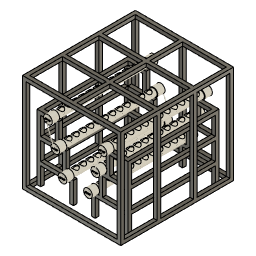
시설 스마트팜 도면 (Autodesk Fusion 360 design; units mm, degrees)
Autodesk Fusion 360 part; units mm, degrees
note: some values were not read from the file. Set by a fixed rule: which face or edge a step refers to.
sketch "스케치1" plane through (0, 0, 0) normal (0, 1, 0) x (1, 0, 0)
  line L0 (0, 0) -> (0, -100)
  line L1 (0, -100) -> (5, -100)
  line L2 (5, -100) -> (5, 0)
  line L3 (5, 0) -> (0, 0)
  dimension "d1" = 100
  dimension "d2" = 5
  constraint vertical L0
  constraint coincident L0.start L3.end
  constraint perpendicular L0 L1
  constraint perpendicular L1 L2
  constraint perpendicular L0 L3
  measures "d1" distance of L0.start L0.end
  measures "d2" distance of L0.end L1.end
extrude "돌출1" add sketch "스케치1" along normal blind 5 makes body 1
copy_body "CopyPasteBodies1" bodies 1 makes body 2
move_body "이동1" bodies 2 to x (1, 0, 0) y (0, 1, 0) z (0, 0, 1) at (70, 0, 0)
copy_body "CopyPasteBodies2" bodies 1 makes body 3
move_body "이동2" bodies 3 to x (0, 0, 1) y (0, 1, 0) z (-1, 0, 0) at (100, 0, 100)
extrude "돌출2" cut 1 faces at (100, 1.6667, 103.3333) along direction (-1, 0, 0) blind 25 on bodies 3 bodies 3
copy_body "CopyPasteBodies3" bodies 1 2 3 makes body 4 makes body 5 makes body 6
move_body "이동3" bodies 4 5 6 to x (1, 0, 0) y (0, 1, 0) z (0, 0, 1) at (0, 50, 0)
copy_body "CopyPasteBodies4" bodies 4 6 5 makes body 7 makes body 8 makes body 9
move_body "이동4" bodies 7 8 9 to x (1, 0, 0) y (0, 1, 0) z (0, 0, 1) at (0, 50, 0)
copy_body "CopyPasteBodies5" bodies 7 8 9 makes body 10 makes body 11 makes body 12
move_body "이동5" bodies 10 11 12 to x (1, 0, 0) y (0, 1, 0) z (0, 0, 1) at (0, 50, 0)
copy_body "CopyPasteBodies6" bodies 1 makes body 13
move_body "이동6" bodies 13 to x (1, 0, 0) y (0, 0, 1) z (0, -1, 0) at (0, 100, 100)
extrude "돌출3" cut 2 faces at (0, 51.6667, 101.6667) (0, 101.6667, 101.6667) along direction (1, 0, 0) blind 5 on bodies 6 8 bodies 6 8
extrude "돌출4" cut 2 faces at (75, 51.6667, 103.3333) (75, 101.6667, 103.3333) along direction (-1, 0, 0) blind 5 on bodies 6 8 bodies 6 8
move_body "이동7" bodies 13 to x (1, 0, 0) y (0, 1, 0) z (0, 0, 1) at (0, 5, 0)
extrude "돌출5" add 1 faces at (3.3333, 105, 103.3333) along direction (0, 1, 0) blind 45 on bodies 13 bodies 13
copy_body "CopyPasteBodies7" bodies 13 makes body 14
move_body "이동8" bodies 14 to x (1, 0, 0) y (0, 1, 0) z (0, 0, 1) at (70, 0, 0)
combine "결합1" operation add target body 1 tool bodies 2 3 4 5 6 7 8 9 10 11 12 13 14
extrude "돌출6" add 1 faces at (75, 85, 103.3333) along direction (1, 0, 0) blind 15 on bodies 1 bodies 1
extrude "돌출7" cut 7 faces at (70, 3.3333, 66.6667) (70, 51.6667, 33.3333) (70, 101.6667, 33.3333) (70, 151.6667, 33.3333) (70, 135, 101.6667) (70, 85, 101.6667) (70, 20, 101.6667) along direction (1, 0, 0) blind 15 on bodies 1 bodies 1
sketch "스케치2" plane through (0, 0, 0) normal (0, -1, 0) x (1, 0, 0)
  line L0 (5, 100) -> (85, 100)
  line L1 (85, 100) -> (85, 0)
  line L2 (85, 0) -> (90, 0)
  line L3 (90, 0) -> (90, 105)
  line L4 (90, 105) -> (0, 105)
  line L5 (0, 105) -> (0, 0)
  line L6 (0, 0) -> (5, 0)
  line L7 (5, 0) -> (5, 100)
  line L8 (42.5, 105) -> (42.5, 100)
  line L9 (47.5, 100) -> (47.5, 105)
  dimension "d18" = 5
  constraint coincident L0 L8.end
  constraint perpendicular L0 L8
  constraint coincident L4 L9.end
  constraint perpendicular L4 L9
  measures "d18" distance of L8.end L9.start
extrude "돌출8" add sketch "스케치2" against normal blind 155 contours L0 L4 L8 L9 bodies 1
sketch "스케치3" plane through (0, 0, 0) normal (-1, 0, 0) x (0, -1, 0)
  line L0 (-100, 0) -> (-100, 100)
  line L1 (-100, 100) -> (-55, 100)
  line L2 (-55, 100) -> (-55, 0)
  line L3 (-55, 0) -> (-50, 0)
  line L4 (-50, 0) -> (-50, 100)
  line L5 (-50, 100) -> (-5, 100)
  line L6 (-5, 100) -> (-5, 0)
  line L7 (-5, 0) -> (0, 0)
  line L8 (0, 0) -> (0, 105)
  line L9 (0, 105) -> (-155, 105)
  line L10 (-155, 105) -> (-155, 0)
  line L11 (-155, 0) -> (-150, 0)
  line L12 (-150, 0) -> (-150, 100)
  line L13 (-150, 100) -> (-105, 100)
  line L14 (-105, 100) -> (-105, 0)
  line L15 (-105, 0) -> (-100, 0)
  line L16 (-155, 0) -> (0, 0)
  line L17 (0, 0) -> (0, 5)
  line L18 (0, 5) -> (-155, 5)
  dimension "d21" = 5
  constraint coincident L10.end L11.start
  constraint coincident L7.end L8.start
  constraint coincident L8 L17.end
  constraint coincident L10 L18.end
  constraint perpendicular L10 L18
  measures "d21" distance of L7.end L17.end
extrude "돌출9" add sketch "스케치3" against normal blind 5 contours L0 L2 L16 L18 | L12 L14 L16 L18 | L4 L6 L16 L18 bodies 1
extrude "돌출10" add sketch "스케치3" against normal blind 85 contours L6 L7 L8 L16 L17 L18 bodies 1
extrude "돌출11" add sketch "스케치3" against normal blind 85 contours L10 L11 L12 L16 L18 bodies 1
extrude "돌출12" add sketch "스케치3" along normal blind -85 and the other way blind 90 contours L0 L2 L16 L18 | L12 L14 L16 L18 | L4 L6 L16 L18 bodies 1
extrude "돌출13" add 1 faces at (90, 85, 103.3333) along direction (1, 0, 0) blind 30 on bodies 1 bodies 1
extrude "돌출14" cut 6 faces at (85, 1.6667, 68.3333) (85, 70, 1.6667) (85, 153.3333, 36.6667) (85, 20, 101.6667) (85, 85, 101.6667) (85, 135, 101.6667) along direction (1, 0, 0) blind 30 on bodies 1 bodies 1
extrude "돌출15" add 3 faces at (47.5, 20, 101.6667) (47.5, 70, 101.6667) (47.5, 120, 101.6667) along direction (1, 0, 0) blind 15 on bodies 1 bodies 1
extrude "돌출16" cut 3 faces at (42.5, 20, 101.6667) (42.5, 70, 103.3333) (42.5, 120, 103.3333) along direction (1, 0, 0) blind 15 on bodies 1 bodies 1
extrude "돌출17" add 1 faces at (118.3333, 85, 105) along direction (0, 0, 1) blind 30 on bodies 1 bodies 1
extrude "돌출18" cut 7 faces at (1.6667, 35, 100) (3.3333, 70, 100) (3.3333, 120, 100) (116.6667, 70, 100) (116.6667, 120, 100) (116.6667, 20, 100) (60.8333, 1.6667, 100) along direction (0, 0, 1) blind 30 on bodies 1 bodies 1
sketch "스케치4" plane through (0, 0, 0) normal (0, 1, 0) x (1, 0, 0)
  line L0 (5, -90) -> (25, -90)
  line L1 (45, 0) -> (5, 0)
  line L2 (5, 0) -> (5, -90)
  circle A0 centre (42.5, -32.5) radius 2.5
  line L3 (10, -55) -> (35, -55)
  line L4 (35, -55) -> (35, -30)
  line L5 (35, -30) -> (10, -30)
  line L6 (10, -30) -> (10, -55)
  circle A1 centre (37.5, -62.5) radius 2.5
  line L7 (10, -85) -> (30, -85)
  line L8 (30, -85) -> (30, -60)
  line L9 (30, -60) -> (10, -60)
  line L10 (10, -60) -> (10, -85)
  line L11 (25, -90) -> (35, -90)
  line L12 (35, -90) -> (35, -60)
  line L13 (35, -60) -> (40, -60)
  line L14 (40, -60) -> (40, -30)
  line L15 (40, -30) -> (45, -30)
  line L16 (45, -30) -> (45, 0)
  line L17 (10, 0) -> (10, -25)
  line L18 (10, -25) -> (40, -25)
  line L19 (40, -25) -> (40, 0)
  circle A2 centre (32.5, -92.5) radius 2.5
  dimension "d63" = 90
  dimension "d77" = 20
  dimension "d78" = 25
  dimension "d80" = 25
  dimension "d82" = 25
  dimension "d83" = 30
  constraint perpendicular L1 L2
  constraint horizontal L3
  constraint vertical L4
  constraint horizontal L5
  constraint vertical L6
  constraint horizontal L7
  constraint vertical L8
  constraint horizontal L9
  constraint vertical L10
  constraint perpendicular L12 L13
  constraint perpendicular L15 L16
  constraint perpendicular L17 L18
  constraint coincident L1 L19.end
  constraint perpendicular L1 L19
  measures "d63" distance of L0 L1
  measures "d77" distance of L7.start L7.end
  measures "d78" distance of L3.start L3.end
  measures "d80" distance of L3.start L5.end
  measures "d82" distance of L17.start L17.end
  measures "d83" distance of L17.end L18.end
extrude "돌출19" add sketch "스케치4" along normal blind 10 and the other way blind -5 separate body contours L0 L1 L2 L11 L12 L13 L14 L15 L16 L17 L18 L19 makes body 15
sketch "스케치5" plane through (0, 5, 0) normal (0, -1, 0) x (1, 0, 0)
  line L0 (10, 60) -> (10, 85)
  line L1 (10, 85) -> (30, 85)
  line L2 (30, 85) -> (30, 60)
  line L3 (30, 60) -> (10, 60)
  line L4 (10, 30) -> (10, 55)
  line L5 (10, 55) -> (35, 55)
  line L6 (35, 55) -> (35, 30)
  line L7 (35, 30) -> (10, 30)
  line L8 (5, 0) -> (10, 0)
  line L9 (10, 0) -> (10, 25)
  line L10 (10, 25) -> (40, 25)
  line L11 (40, 25) -> (40, 0)
  line L12 (40, 0) -> (45, 0)
  line L13 (45, 0) -> (45, 30)
  line L14 (45, 30) -> (40, 30)
  line L15 (40, 30) -> (40, 60)
  line L16 (40, 60) -> (35, 60)
  line L17 (35, 60) -> (35, 90)
  line L18 (35, 90) -> (5, 90)
  line L19 (5, 90) -> (5, 0)
  line L20 (10, 60) -> (5, 60)
  line L21 (5, 60) -> (5, 55)
  line L22 (5, 55) -> (10, 55)
  line L23 (10, 55) -> (10, 60)
  line L24 (10, 30) -> (5, 30)
  line L25 (5, 30) -> (5, 25)
  line L26 (5, 25) -> (10, 25)
  line L27 (10, 25) -> (10, 30)
  line L28 (10, 85) -> (5, 85)
  line L29 (5, 85) -> (5, 90)
  line L30 (5, 90) -> (10, 90)
  line L31 (10, 90) -> (10, 85)
  constraint horizontal L20
  constraint vertical L21
  constraint horizontal L22
  constraint vertical L23
  constraint coincident L19 L21.end
  constraint coincident L0.start L3.end
  constraint horizontal L24
  constraint vertical L25
  constraint horizontal L26
  constraint vertical L27
  constraint coincident L19 L25.end
  constraint coincident L4.start L7.end
  constraint horizontal L28
  constraint vertical L29
  constraint horizontal L30
  constraint vertical L31
  constraint coincident L18.end L19.start
  constraint coincident L0.end L1.start
extrude "돌출20" add sketch "스케치5" against normal blind 145 contours L19 L20 L21 L22 L23 | L18 L19 L28 L29 L30 L31 | L19 L24 L25 L26 L27 bodies 15
extrude "돌출21" add 4 faces at (6.6667, 10, 68.3333) (6.6667, 10, 38.3333) (6.6667, 10, 8.3333) (33.3333, 10, 78.3333) along direction (0, 1, 0) blind 140 and the other way blind -135 on bodies 15 bodies 15
extrude "돌출22" add 2 faces at (45, 6.6667, 20) (45, 146.6667, 20) along direction (1, 0, 0) blind 10 on bodies 15 bodies 15
extrude "돌출23" cut 2 faces at (40, 6.6667, 16.6667) (40, 146.6667, 16.6667) along direction (1, 0, 0) blind 10 on bodies 15 bodies 15
extrude "돌출24" add 2 faces at (40, 6.6667, 50) (40, 146.6667, 50) along direction (1, 0, 0) blind 5 on bodies 15 bodies 15
extrude "돌출25" cut 2 faces at (35, 146.6667, 46.6667) (35, 6.6667, 46.6667) along direction (1, 0, 0) blind 5 on bodies 15 bodies 15
sketch "스케치6" plane through (0, 5, 0) normal (0, -1, 0) x (1, 0, 0)
  line L0 (10, 85) -> (30, 85)
  line L1 (30, 85) -> (30, 60)
  line L2 (30, 60) -> (10, 60)
  line L3 (10, 60) -> (10, 85)
  line L4 (10, 55) -> (40, 55)
  line L5 (40, 55) -> (40, 30)
  line L6 (40, 30) -> (10, 30)
  line L7 (10, 30) -> (10, 55)
  line L8 (10, 25) -> (50, 25)
  line L9 (50, 25) -> (50, 0)
  line L10 (50, 0) -> (55, 0)
  line L11 (55, 0) -> (55, 30)
  line L12 (55, 30) -> (45, 30)
  line L13 (45, 30) -> (45, 60)
  line L14 (45, 60) -> (35, 60)
  line L15 (35, 60) -> (35, 90)
  line L16 (35, 90) -> (5, 90)
  line L17 (5, 90) -> (5, 0)
  line L18 (5, 0) -> (10, 0)
  line L19 (10, 0) -> (10, 25)
  circle A0 centre (40, 65) radius 5
  line L20 (35, 90) -> (30, 90)
  circle A1 centre (30, 95) radius 5
  circle A2 centre (50, 35) radius 5
  constraint coincident L15.end L16.start
  constraint perpendicular L15 L20
  constraint coincident L20.end A1
copy_body "CopyPasteBodies8" bodies 15 makes body 16
move_body "이동9" bodies 16 to x (-1, 0, 0) y (0, -1, 0) z (0, 0, 1) at (120, 155, 0)
extrude "돌출26" add 1 faces at (120, 85, 133.3333) along direction (1, 0, 0) blind 15 on bodies 1 bodies 1
extrude "돌출27" cut 6 faces at (115, 1.6667, 88.3333) (115, 70, 1.6667) (115, 151.6667, 46.6667) (115, 20, 131.6667) (115, 85, 131.6667) (115, 135, 133.3333) along direction (1, 0, 0) blind 15 on bodies 1 bodies 1
extrude "돌출28" add 3 faces at (62.5, 20, 131.6667) (62.5, 70, 131.6667) (62.5, 120, 131.6667) along direction (1, 0, 0) blind 7.5 on bodies 1 bodies 1
extrude "돌출29" cut 3 faces at (57.5, 20, 131.6667) (57.5, 70, 131.6667) (57.5, 120, 131.6667) along direction (1, 0, 0) blind 7.5 on bodies 1 bodies 1
move_body "이동10" bodies 16 to x (1, 0, 0) y (0, 1, 0) z (0, 0, 1) at (15, 0, 0)
extrude "돌출30" add sketch "스케치6" against normal blind 145 separate body contours A1 | A2 | A0 makes body 17 at (34.9752, 101.6667, 94.5022) makes body 18 at (44.9752, 53.3333, 65.4978) makes body 19 at (54.9752, 53.3333, 35.4978)
extrude "돌출31" add 8 faces at (6.6667, 10, 8.3333) (6.6667, 10, 38.3333) (6.6667, 10, 68.3333) (33.3333, 10, 26.6667) (128.3333, 10, 8.3333) (128.3333, 10, 38.3333) (128.3333, 10, 68.3333) (101.6667, 10, 26.6667) along direction (0, 1, 0) blind 10 on bodies 15 16 bodies 15 16
extrude "돌출32" cut 2 faces at (6.6667, 5, 50) (128.3333, 5, 40) along direction (0, 1, 0) blind 10 on bodies 15 16 bodies 15 16
extrude "돌출33" add 8 faces at (6.6667, 145, 8.3333) (6.6667, 145, 38.3333) (6.6667, 145, 68.3333) (33.3333, 145, 26.6667) (128.3333, 145, 16.6667) (128.3333, 145, 38.3333) (128.3333, 145, 68.3333) (101.6667, 145, 26.6667) along direction (0, -1, 0) blind 10 on bodies 15 16 bodies 15 16
extrude "돌출34" cut 2 faces at (128.3333, 150, 50) (6.6667, 150, 40) along direction (0, -1, 0) blind 10 on bodies 15 16 bodies 15 16
shell "쉘1" thickness 1 removed faces 3 at (31.4276, 5, 95.2319) at (41.4462, 5, 64.9835) at (49.3001, 5, 32.2341) on bodies 17 18 19
extrude "돌출35" cut 3 faces at (31.1017, 149, 95.7511) (41.146, 149, 65.9454) (48.7702, 149, 34.8013) along direction (0, 1, 0) blind 50 on bodies 17 18 19 bodies 17 18 19
sketch "스케치7" plane through (0, 5, 0) normal (0, -1, 0) x (1, 0, 0)
  circle A0 centre (30, 95) radius 4
  circle A1 centre (30, 95) radius 5
  circle A2 centre (30, 95) radius 6
  dimension "d130" = 12
  constraint concentric A0 A2
  measures "d130" diameter of A2
extrude "돌출36" add sketch "스케치7" against normal blind 10 contours A2 bodies 17
extrude "돌출37" add sketch "스케치7" against normal blind 1 contours A0 bodies 17
extrude "돌출38" add sketch "스케치7" along normal blind -145 and the other way blind 135 contours A2 bodies 17
extrude "돌출39" add sketch "스케치7" along normal blind -145 and the other way blind 144 contours A0 bodies 17
sketch "스케치8" plane through (0, 5, 0) normal (0, -1, 0) x (1, 0, 0)
  circle A0 centre (40, 65) radius 4
  circle A1 centre (40, 65) radius 5
  circle A2 centre (40, 65) radius 6
  dimension "d143" = 12
  constraint concentric A0 A2
  measures "d143" diameter of A2
extrude "돌출40" add sketch "스케치8" against normal blind 10 contours A2 bodies 18
extrude "돌출41" add sketch "스케치8" against normal blind 1 contours A0 bodies 18
extrude "돌출42" add sketch "스케치8" along normal blind -145 and the other way blind 135 contours A2 bodies 18
extrude "돌출43" add sketch "스케치8" along normal blind -145 and the other way blind 144 contours A0 bodies 18
sketch "스케치9" plane through (0, 5, 0) normal (0, -1, 0) x (1, 0, 0)
  circle A0 centre (50, 35) radius 4
  circle A1 centre (50, 35) radius 5
  circle A2 centre (50, 35) radius 6
  dimension "d156" = 12
  constraint concentric A0 A2
  measures "d156" diameter of A2
extrude "돌출44" add sketch "스케치9" against normal blind 10 contours A2 bodies 19
extrude "돌출45" add sketch "스케치9" against normal blind 1 contours A0 bodies 19
extrude "돌출46" add sketch "스케치9" along normal blind -145 and the other way blind 135 contours A2 bodies 19
extrude "돌출47" add sketch "스케치9" along normal blind -145 and the other way blind 144 contours A0 bodies 19
copy_body "CopyPasteBodies9" bodies 17 makes body 20
move_body "이동11" bodies 20 to x (1, 0, 0) y (0, 1, 0) z (0, 0, 1) at (75, 0, 0)
copy_body "CopyPasteBodies10" bodies 18 makes body 21
move_body "이동12" bodies 21 to x (1, 0, 0) y (0, 1, 0) z (0, 0, 1) at (55, 0, 0)
copy_body "CopyPasteBodies11" bodies 19 makes body 22
move_body "이동13" bodies 22 to x (1, 0, 0) y (0, 1, 0) z (0, 0, 1) at (35, 0, 0)
sketch "스케치10" plane through (0, 0, 90) normal (0, 0, 1) x (-1, 0, 0)
  line L0 (-35, -140) -> (-5, -140)
  line L1 (-5, -140) -> (-5, -15)
  line L2 (-5, -15) -> (-35, -15)
  line L3 (-35, -15) -> (-35, -20)
  line L4 (-35, -20) -> (-10, -20)
  line L5 (-10, -20) -> (-10, -135)
  line L6 (-10, -135) -> (-35, -135)
  line L7 (-35, -135) -> (-35, -140)
  line L8 (-35, -140) -> (-25, -140)
  circle A0 centre (-30, -132.5) radius 4
  circle A1 centre (-30, -122.5) radius 4
  circle A2 centre (-30, -112.5) radius 4
  circle A3 centre (-30, -102.5) radius 4
  circle A4 centre (-30, -92.5) radius 4
  circle A5 centre (-30, -82.5) radius 4
  circle A6 centre (-30, -72.5) radius 4
  circle A7 centre (-30, -62.5) radius 4
  circle A8 centre (-30, -52.5) radius 4
  circle A9 centre (-30, -42.5) radius 4
  circle A10 centre (-30, -32.5) radius 4
  circle A11 centre (-30, -22.5) radius 4
  circle A12 centre (-40, -132.5) radius 4
  circle A13 centre (-40, -122.5) radius 4
  circle A14 centre (-40, -112.5) radius 4
  circle A15 centre (-40, -102.5) radius 4
  circle A16 centre (-40, -92.5) radius 4
  circle A17 centre (-40, -82.5) radius 4
  circle A18 centre (-40, -72.5) radius 4
  circle A19 centre (-40, -62.5) radius 4
  circle A20 centre (-40, -52.5) radius 4
  circle A21 centre (-40, -42.5) radius 4
  circle A22 centre (-40, -32.5) radius 4
  circle A23 centre (-40, -22.5) radius 4
  circle A24 centre (-50, -132.5) radius 4
  circle A25 centre (-50, -122.5) radius 4
  circle A26 centre (-50, -112.5) radius 4
  circle A27 centre (-50, -102.5) radius 4
  circle A28 centre (-50, -92.5) radius 4
  circle A29 centre (-50, -82.5) radius 4
  circle A30 centre (-50, -72.5) radius 4
  circle A31 centre (-50, -62.5) radius 4
  circle A32 centre (-50, -52.5) radius 4
  circle A33 centre (-50, -42.5) radius 4
  circle A34 centre (-50, -32.5) radius 4
  circle A35 centre (-50, -22.5) radius 4
  dimension "d169" = 10
  dimension "d171" = 8
  dimension "d172" = 8
  dimension "d173" = 8
  dimension "d174" = 8
  dimension "d175" = 8
  dimension "d176" = 8
  dimension "d177" = 8
  dimension "d178" = 8
  dimension "d179" = 8
  dimension "d180" = 8
  dimension "d181" = 8
  dimension "d182" = 8
  dimension "d183" = 8
  dimension "d184" = 8
  dimension "d185" = 8
  dimension "d186" = 8
  dimension "d187" = 8
  dimension "d188" = 8
  dimension "d189" = 8
  dimension "d190" = 8
  dimension "d191" = 8
  dimension "d192" = 8
  dimension "d193" = 8
  dimension "d194" = 8
  dimension "d195" = 8
  dimension "d196" = 8
  dimension "d197" = 8
  dimension "d198" = 8
  dimension "d199" = 8
  dimension "d200" = 8
  dimension "d201" = 8
  dimension "d202" = 8
  dimension "d203" = 8
  dimension "d204" = 8
  dimension "d205" = 8
  dimension "d206" = 8
  constraint coincident L0.start L7.end
  constraint perpendicular L7 L8
  measures "d169" distance of L0.start L8.end
  measures "d171" diameter of A0
  measures "d172" diameter of A1
  measures "d173" diameter of A2
  measures "d174" diameter of A3
  measures "d175" diameter of A4
  measures "d176" diameter of A5
  measures "d177" diameter of A6
  measures "d178" diameter of A7
  measures "d179" diameter of A8
  measures "d180" diameter of A9
  measures "d181" diameter of A10
  measures "d182" diameter of A11
  measures "d183" diameter of A12
  measures "d184" diameter of A13
  measures "d185" diameter of A14
  measures "d186" diameter of A15
  measures "d187" diameter of A16
  measures "d188" diameter of A17
  measures "d189" diameter of A18
  measures "d190" diameter of A19
  measures "d191" diameter of A20
  measures "d192" diameter of A21
  measures "d193" diameter of A22
  measures "d194" diameter of A23
  measures "d195" diameter of A24
  measures "d196" diameter of A25
  measures "d197" diameter of A26
  measures "d198" diameter of A27
  measures "d199" diameter of A28
  measures "d200" diameter of A29
  measures "d201" diameter of A30
  measures "d202" diameter of A31
  measures "d203" diameter of A32
  measures "d204" diameter of A33
  measures "d205" diameter of A34
  measures "d206" diameter of A35
extrude "돌출48" cut sketch "스케치10" along normal blind 10 and the other way blind -5 contours L6 A0 | L6 A0 | L4 A11 | L4 A11 | A1 | A2 | A3 | A4 | A5 | A6 | A7 | A8 | A9 | A10 bodies 17
extrude "돌출49" cut sketch "스케치10" against normal blind 25 contours A12 | A13 | A14 | A15 | A16 | A17 | A18 | A19 | A20 | A21 | A22 | A23 bodies 18
extrude "돌출50" cut sketch "스케치10" against normal blind 55 contours A24 | A25 | A26 | A27 | A28 | A29 | A30 | A31 | A32 | A33 | A34 | A35 bodies 19
move_body "이동14" bodies 20 21 22 to x (1, 0, 0) y (0, 1, 0) z (0, 0, 1) at (-55, 0, 0)
extrude "돌출51" cut sketch "스케치10" along normal blind 10 and the other way blind -5 contours A24 | A25 | A26 | A27 | A28 | A29 | A30 | A31 | A32 | A33 | A34 | A35 bodies 20
extrude "돌출52" cut sketch "스케치10" against normal blind 25 contours A12 | A13 | A14 | A15 | A16 | A17 | A18 | A19 | A20 | A21 | A22 | A23 bodies 21
extrude "돌출53" cut sketch "스케치10" against normal blind 55 contours L6 A0 | L6 A0 | L4 A11 | L4 A11 | A1 | A2 | A3 | A4 | A5 | A6 | A7 | A8 | A9 | A10 bodies 22
move_body "이동15" bodies 20 21 22 to x (1, 0, 0) y (0, 1, 0) z (0, 0, 1) at (55, 0, 0)
sketch "스케치11" plane through (0, 5, 0) normal (0, -1, 0) x (1, 0, 0)
  circle A0 centre (30, 95) radius 6
  line L0 (28.75, 95.5) -> (26.75, 95.5)
  line L1 (26.25, 95) -> (26.25, 95)
  line L2 (26.75, 94.5) -> (28.75, 94.5)
  line L3 (29.25, 95) -> (29.25, 95)
  line L4 (33.25, 94.5) -> (31.25, 94.5)
  line L5 (30.75, 95) -> (30.75, 95)
  line L6 (33.75, 95) -> (33.75, 95)
  line L7 (31.25, 95.5) -> (33.25, 95.5)
  arc A1 (26.75, 95.5) -> (26.25, 95) centre (26.75, 95) ccw
  arc A2 (26.25, 95) -> (26.75, 94.5) centre (26.75, 95) ccw
  arc A3 (29.25, 95) -> (28.75, 95.5) centre (28.75, 95) ccw
  arc A4 (28.75, 94.5) -> (29.25, 95) centre (28.75, 95) ccw
  arc A5 (31.25, 95.5) -> (30.75, 95) centre (31.25, 95) ccw
  arc A6 (30.75, 95) -> (31.25, 94.5) centre (31.25, 95) ccw
  arc A7 (33.75, 95) -> (33.25, 95.5) centre (33.25, 95) ccw
  arc A8 (33.25, 94.5) -> (33.75, 95) centre (33.25, 95) ccw
  constraint tangent L0 A1
  constraint tangent L2 A2
  constraint tangent L0 A3
  constraint tangent L2 A4
  constraint tangent L7 A5
  constraint tangent L4 A6
  constraint tangent L7 A7
  constraint tangent L4 A8
extrude "돌출54" add sketch "스케치11" along normal blind 1 contours L0 L2 A1 A2 A3 A4 | L4 L7 A5 A6 A7 A8 bodies 17
fillet "모깎기1" radius 0.1 8 edges at (32.25, 4, 94.5) (33.75, 4, 95) (32.25, 4, 95.5) (30.75, 4, 95) (27.75, 4, 94.5) (29.25, 4, 95) (27.75, 4, 95.5) (26.25, 4, 95) on bodies 17
sketch "스케치12" plane through (0, 0, 0) normal (1, 0, 0) x (0, 1, 0)
  line L0 (0, 0) -> (0, 2.5045)
  line L1 (0, 95.0045) -> (-1, 95.0045)
  line L2 (-2, 94.0045) -> (-2, 93.0045)
  arc A0 (-1, 95.0045) -> (-2, 94.0045) centre (-1, 94.0045) ccw
  point P0 (-2, 95.0045)
  dimension "d239" = 92.5
  dimension "d240" = 2
  dimension "d241" = 2
  dimension "d242" = 1
  constraint coincident L0.start origin
  constraint vertical L0
  constraint perpendicular L1 L2
  constraint coincident P0 L1
  constraint coincident P0 L2
  constraint tangent L1 A0
  constraint tangent L2 A0
  measures "d239" distance of L0.end L1.start
  measures "d240" distance of L1.start P0
  measures "d241" distance of P0 L2.end
  measures "d242" radius of A0
pipe "파이프1" add diameter 1 path "스케치12" along L1 A0 L2 separate body makes body 23
move_body "이동16" bodies 23 to x (1, 0, 0) y (0, 1, 0) z (0, 0, 1) at (30, 4.8, 0)
sketch "스케치13" plane through (0, 5, 0) normal (0, -1, 0) x (1, 0, 0)
  circle A0 centre (40, 65) radius 6
  line L0 (38.75, 65.5) -> (36.75, 65.5)
  arc A1 (36.75, 65.5) -> (36.75, 64.5) centre (36.75, 65) ccw
  line L1 (36.75, 64.5) -> (38.75, 64.5)
  arc A2 (38.75, 64.5) -> (38.75, 65.5) centre (38.75, 65) ccw
  line L2 (38.75, 65) -> (36.75, 65) construction
  line L3 (41.25, 64.5) -> (43.25, 64.5)
  arc A3 (43.25, 64.5) -> (43.25, 65.5) centre (43.25, 65) ccw
  line L4 (43.25, 65.5) -> (41.25, 65.5)
  arc A4 (41.25, 65.5) -> (41.25, 64.5) centre (41.25, 65) ccw
  line L5 (41.25, 65) -> (43.25, 65) construction
  point P0 (36.25, 65.5)
  point P1 (39.25, 64.5)
  constraint tangent L0 A1
  constraint tangent A1 L1
  constraint parallel L0 L1
  constraint tangent L1 A2
  constraint tangent L0 A2
  constraint horizontal L2
  constraint tangent L3 A3
  constraint tangent A3 L4
  constraint parallel L3 L4
  constraint tangent L4 A4
  constraint tangent L3 A4
extrude "돌출55" add sketch "스케치13" along normal blind 1 contours L0 A1 L1 A2 | L3 A3 L4 A4 bodies 18
fillet "모깎기2" radius 0.1 8 edges at (37.75, 4, 64.5) (39.25, 4, 65) (37.75, 4, 65.5) (36.25, 4, 65) (42.25, 4, 64.5) (43.75, 4, 65) (42.25, 4, 65.5) (40.75, 4, 65) on bodies 18
copy_body "CopyPasteBodies12" bodies 23 makes body 24
move_body "이동17" bodies 24 to x (-1, 0, 0) y (0, 1, 0) z (0, 0, -1) at (70, 0.2, 160.0089)
move_body "이동18" bodies 23 to x (1, 0, 0) y (0, 1, 0) z (0, 0, 1) at (0, 0.2, 0)
copy_body "CopyPasteBodies13" bodies 23 makes body 25
move_body "이동19" bodies 25 to x (-1, 0, 0) y (0, -1, 0) z (0, 0, 1) at (60, 155, 0)
sketch "스케치14" plane through (0, 150, 0) normal (0, 1, 0) x (-1, 0, 0)
  circle A0 centre (-30, 95) radius 6
  line L0 (-33.25, 94.5) -> (-31.25, 94.5)
  arc A1 (-31.25, 94.5) -> (-31.25, 95.5) centre (-31.25, 95) ccw
  line L1 (-31.25, 95.5) -> (-33.25, 95.5)
  arc A2 (-33.25, 95.5) -> (-33.25, 94.5) centre (-33.25, 95) ccw
  line L2 (-33.25, 95) -> (-31.25, 95) construction
  arc A3 (-26.75, 94.5) -> (-26.75, 95.5) centre (-26.75, 95) ccw
  line L3 (-26.75, 94.5) -> (-28.75, 94.5)
  line L4 (-28.75, 95.5) -> (-26.75, 95.5)
  arc A4 (-28.75, 95.5) -> (-28.75, 94.5) centre (-28.75, 95) ccw
  point P0 (-33.75, 95.5)
  constraint tangent L0 A1
  constraint tangent A1 L1
  constraint parallel L0 L1
  constraint tangent L1 A2
  constraint tangent L0 A2
extrude "돌출56" add sketch "스케치14" along normal blind 1 contours L0 A1 L1 A2 | A3 L3 L4 A4 bodies 17
fillet "모깎기3" radius 0.1 8 edges at (32.25, 151, 94.5) (30.75, 151, 95) (32.25, 151, 95.5) (33.75, 151, 95) (27.75, 151, 94.5) (26.25, 151, 95) (27.75, 151, 95.5) (29.25, 151, 95) on bodies 17
sketch "스케치15" plane through (0, 150, 0) normal (0, 1, 0) x (-1, 0, 0)
  circle A0 centre (-40, 65) radius 6
  line L0 (-43.25, 64.5) -> (-41.25, 64.5)
  arc A1 (-41.25, 64.5) -> (-41.25, 65.5) centre (-41.25, 65) ccw
  line L1 (-41.25, 65.5) -> (-43.25, 65.5)
  arc A2 (-43.25, 65.5) -> (-43.25, 64.5) centre (-43.25, 65) ccw
  line L2 (-43.25, 65) -> (-41.25, 65) construction
  line L3 (-36.75, 64.5) -> (-38.75, 64.5)
  arc A3 (-38.75, 65.5) -> (-38.75, 64.5) centre (-38.75, 65) ccw
  arc A4 (-36.75, 64.5) -> (-36.75, 65.5) centre (-36.75, 65) ccw
  line L4 (-38.75, 65.5) -> (-36.75, 65.5)
  point P0 (-43.75, 65.5)
  point P1 (-40.75, 64.5)
  constraint tangent L0 A1
  constraint tangent A1 L1
  constraint parallel L0 L1
  constraint tangent L1 A2
  constraint tangent L0 A2
  constraint horizontal L2
extrude "돌출57" add sketch "스케치15" along normal blind 1 contours L0 A1 L1 A2 | L3 A3 A4 L4 bodies 18
fillet "모깎기4" radius 0.1 8 edges at (42.25, 151, 64.5) (40.75, 151, 65) (42.25, 151, 65.5) (43.75, 151, 65) (36.25, 151, 65) (37.75, 151, 65.5) (39.25, 151, 65) (37.75, 151, 64.5) on bodies 18
copy_body "CopyPasteBodies14" bodies 25 makes body 26
move_body "이동20" bodies 26 to x (1, 0, 0) y (0, 1, 0) z (0, 0, 1) at (10, 0, -30)
sketch "스케치16" plane through (0, 5, 0) normal (0, -1, 0) x (1, 0, 0)
  circle A0 centre (50, 35) radius 6
  line L0 (46.75, 34.5) -> (48.75, 34.5)
  arc A1 (48.75, 34.5) -> (48.75, 35.5) centre (48.75, 35) ccw
  line L1 (48.75, 35.5) -> (46.75, 35.5)
  arc A2 (46.75, 35.5) -> (46.75, 34.5) centre (46.75, 35) ccw
  line L2 (46.75, 35) -> (48.75, 35) construction
  line L3 (53.25, 34.5) -> (51.25, 34.5)
  arc A3 (51.25, 35.5) -> (51.25, 34.5) centre (51.25, 35) ccw
  arc A4 (53.25, 34.5) -> (53.25, 35.5) centre (53.25, 35) ccw
  line L4 (51.25, 35.5) -> (53.25, 35.5)
  point P0 (46.25, 35.5)
  constraint tangent L0 A1
  constraint tangent A1 L1
  constraint parallel L0 L1
  constraint tangent L1 A2
  constraint tangent L0 A2
extrude "돌출58" add sketch "스케치16" along normal blind 1 contours L0 A1 L1 A2 | L3 A3 A4 L4 bodies 19
fillet "모깎기5" radius 0.1 8 edges at (52.25, 4, 34.5) (53.75, 4, 35) (52.25, 4, 35.5) (50.75, 4, 35) (47.75, 4, 34.5) (49.25, 4, 35) (47.75, 4, 35.5) (46.25, 4, 35) on bodies 19
copy_body "CopyPasteBodies15" bodies 24 makes body 27
move_body "이동21" bodies 27 to x (1, 0, 0) y (0, 1, 0) z (0, 0, 1) at (10, 0, -30)
copy_body "CopyPasteBodies16" bodies 27 makes body 28
move_body "이동22" bodies 28 to x (-1, 0, 0) y (0, -1, 0) z (0, 0, 1) at (100, 155, 0)
sketch "스케치17" plane through (0, 150, 0) normal (0, 1, 0) x (-1, 0, 0)
  circle A0 centre (-50, 35) radius 6
  line L0 (-53.25, 34.5) -> (-51.25, 34.5)
  arc A1 (-51.25, 34.5) -> (-51.25, 35.5) centre (-51.25, 35) ccw
  line L1 (-51.25, 35.5) -> (-53.25, 35.5)
  arc A2 (-53.25, 35.5) -> (-53.25, 34.5) centre (-53.25, 35) ccw
  line L2 (-53.25, 35) -> (-51.25, 35) construction
  line L3 (-46.75, 34.5) -> (-48.75, 34.5)
  arc A3 (-48.75, 35.5) -> (-48.75, 34.5) centre (-48.75, 35) ccw
  arc A4 (-46.75, 34.5) -> (-46.75, 35.5) centre (-46.75, 35) ccw
  line L4 (-48.75, 35.5) -> (-46.75, 35.5)
  point P0 (-53.75, 35.5)
  constraint tangent L0 A1
  constraint tangent A1 L1
  constraint parallel L0 L1
  constraint tangent L1 A2
  constraint tangent L0 A2
  constraint horizontal L2
extrude "돌출59" add sketch "스케치17" along normal blind 1 contours L0 A1 L1 A2 | L3 A3 A4 L4 bodies 19
fillet "모깎기6" radius 0.1 8 edges at (52.25, 151, 34.5) (50.75, 151, 35) (52.25, 151, 35.5) (53.75, 151, 35) (47.75, 151, 34.5) (46.25, 151, 35) (47.75, 151, 35.5) (49.25, 151, 35) on bodies 19
combine "결합2" operation add target body 17 tool bodies 23
combine "결합3" operation add target body 17 tool bodies 25
combine "결합4" operation add target body 18 tool bodies 26 24
sketch "스케치18" plane through (0, 5, 0) normal (0, -1, 0) x (1, 0, 0)
  circle A0 centre (105, 95) radius 6
  line L0 (101.75, 94.5) -> (103.75, 94.5)
  arc A1 (103.75, 94.5) -> (103.75, 95.5) centre (103.75, 95) ccw
  line L1 (103.75, 95.5) -> (101.75, 95.5)
  arc A2 (101.75, 95.5) -> (101.75, 94.5) centre (101.75, 95) ccw
  line L2 (101.75, 95) -> (103.75, 95) construction
  line L3 (108.25, 94.5) -> (106.25, 94.5)
  arc A3 (106.25, 95.5) -> (106.25, 94.5) centre (106.25, 95) ccw
  arc A4 (108.25, 94.5) -> (108.25, 95.5) centre (108.25, 95) ccw
  line L4 (106.25, 95.5) -> (108.25, 95.5)
  point P0 (101.25, 95.5)
  constraint tangent L0 A1
  constraint tangent A1 L1
  constraint parallel L0 L1
  constraint tangent L1 A2
  constraint tangent L0 A2
  constraint horizontal L2
sketch "스케치19" plane through (0, 5, 0) normal (0, -1, 0) x (1, 0, 0)
  circle A0 centre (95, 65) radius 6
  line L0 (91.75, 64.5) -> (93.75, 64.5)
  arc A1 (93.75, 64.5) -> (93.75, 65.5) centre (93.75, 65) ccw
  line L1 (93.75, 65.5) -> (91.75, 65.5)
  arc A2 (91.75, 65.5) -> (91.75, 64.5) centre (91.75, 65) ccw
  line L2 (91.75, 65) -> (93.75, 65) construction
  line L3 (98.25, 64.5) -> (96.25, 64.5)
  arc A3 (96.25, 65.5) -> (96.25, 64.5) centre (96.25, 65) ccw
  arc A4 (98.25, 64.5) -> (98.25, 65.5) centre (98.25, 65) ccw
  line L4 (96.25, 65.5) -> (98.25, 65.5)
  point P0 (91.25, 65.5)
  constraint tangent L0 A1
  constraint tangent A1 L1
  constraint parallel L0 L1
  constraint tangent L1 A2
  constraint tangent L0 A2
  constraint horizontal L2
sketch "스케치20" plane through (0, 5, 0) normal (0, -1, 0) x (1, 0, 0)
  circle A0 centre (85, 35) radius 6
  line L0 (81.75, 34.5) -> (83.75, 34.5)
  arc A1 (83.75, 34.5) -> (83.75, 35.5) centre (83.75, 35) ccw
  line L1 (83.75, 35.5) -> (81.75, 35.5)
  arc A2 (81.75, 35.5) -> (81.75, 34.5) centre (81.75, 35) ccw
  line L2 (81.75, 35) -> (83.75, 35) construction
  line L3 (88.25, 34.5) -> (86.25, 34.5)
  arc A3 (86.25, 35.5) -> (86.25, 34.5) centre (86.25, 35) ccw
  arc A4 (88.25, 34.5) -> (88.25, 35.5) centre (88.25, 35) ccw
  line L4 (86.25, 35.5) -> (88.25, 35.5)
  point P0 (81.25, 35.5)
  constraint tangent L0 A1
  constraint tangent A1 L1
  constraint parallel L0 L1
  constraint tangent L1 A2
  constraint tangent L0 A2
  constraint horizontal L2
extrude "돌출60" add sketch "스케치19" sketch "스케치18" sketch "스케치20" along normal blind 1 contours L0 A1 L1 A2 | L3 A3 A4 L4 of sketch 2 contours L0 A1 L1 A2 | L3 A3 A4 L4 of sketch 3 contours L0 A1 L1 A2 | L3 A3 A4 L4 bodies 20 21 22
fillet "모깎기7" radius 0.1 24 edges at (107.25, 4, 95.5) (105.75, 4, 95) (107.25, 4, 94.5) (108.75, 4, 95) (104.25, 4, 95) (102.75, 4, 95.5) (101.25, 4, 95) (102.75, 4, 94.5) (97.25, 4, 65.5) (95.75, 4, 65) (97.25, 4, 64.5) (98.75, 4, 65) (92.75, 4, 65.5) (91.25, 4, 65) (92.75, 4, 64.5) (94.25, 4, 65) (87.25, 4, 35.5) (85.75, 4, 35) (87.25, 4, 34.5) (88.75, 4, 35) (82.75, 4, 35.5) (81.25, 4, 35) (82.75, 4, 34.5) (84.25, 4, 35) on bodies 20 21 22
sketch "스케치21" plane through (0, 150, 0) normal (0, 1, 0) x (-1, 0, 0)
  circle A0 centre (-105, 95) radius 6
  line L0 (-106.25, 95.5) -> (-108.25, 95.5)
  arc A1 (-108.25, 95.5) -> (-108.25, 94.5) centre (-108.25, 95) ccw
  line L1 (-108.25, 94.5) -> (-106.25, 94.5)
  arc A2 (-106.25, 94.5) -> (-106.25, 95.5) centre (-106.25, 95) ccw
  line L2 (-106.25, 95) -> (-108.25, 95) construction
  line L3 (-101.75, 94.5) -> (-103.75, 94.5)
  arc A3 (-103.75, 95.5) -> (-103.75, 94.5) centre (-103.75, 95) ccw
  arc A4 (-101.75, 94.5) -> (-101.75, 95.5) centre (-101.75, 95) ccw
  line L4 (-103.75, 95.5) -> (-101.75, 95.5)
  point P0 (-108.75, 95.5)
  constraint tangent L0 A1
  constraint tangent A1 L1
  constraint parallel L0 L1
  constraint tangent L1 A2
  constraint tangent L0 A2
sketch "스케치22" plane through (0, 150, 0) normal (0, 1, 0) x (-1, 0, 0)
  circle A0 centre (-95, 65) radius 6
  line L0 (-98.25, 64.5) -> (-96.25, 64.5)
  arc A1 (-96.25, 64.5) -> (-96.25, 65.5) centre (-96.25, 65) ccw
  line L1 (-96.25, 65.5) -> (-98.25, 65.5)
  arc A2 (-98.25, 65.5) -> (-98.25, 64.5) centre (-98.25, 65) ccw
  line L2 (-98.25, 65) -> (-96.25, 65) construction
  line L3 (-91.75, 64.5) -> (-93.75, 64.5)
  arc A3 (-93.75, 65.5) -> (-93.75, 64.5) centre (-93.75, 65) ccw
  arc A4 (-91.75, 64.5) -> (-91.75, 65.5) centre (-91.75, 65) ccw
  line L4 (-93.75, 65.5) -> (-91.75, 65.5)
  point P0 (-98.75, 65.5)
  constraint tangent L0 A1
  constraint tangent A1 L1
  constraint parallel L0 L1
  constraint tangent L1 A2
  constraint tangent L0 A2
sketch "스케치23" plane through (0, 150, 0) normal (0, 1, 0) x (-1, 0, 0)
  circle A0 centre (-85, 35) radius 6
  line L0 (-88.25, 34.5) -> (-86.25, 34.5)
  arc A1 (-86.25, 34.5) -> (-86.25, 35.5) centre (-86.25, 35) ccw
  line L1 (-86.25, 35.5) -> (-88.25, 35.5)
  arc A2 (-88.25, 35.5) -> (-88.25, 34.5) centre (-88.25, 35) ccw
  line L2 (-88.25, 35) -> (-86.25, 35) construction
  line L3 (-81.75, 34.5) -> (-83.75, 34.5)
  arc A3 (-83.75, 35.5) -> (-83.75, 34.5) centre (-83.75, 35) ccw
  arc A4 (-81.75, 34.5) -> (-81.75, 35.5) centre (-81.75, 35) ccw
  line L4 (-83.75, 35.5) -> (-81.75, 35.5)
  point P0 (-88.75, 35.5)
  constraint tangent L0 A1
  constraint tangent A1 L1
  constraint parallel L0 L1
  constraint tangent L1 A2
  constraint tangent L0 A2
extrude "돌출61" add sketch "스케치21" sketch "스케치22" sketch "스케치23" along normal blind 1 contours L0 A1 L1 A2 | L3 A3 A4 L4 of sketch 2 contours L0 A1 L1 A2 | L3 A3 A4 L4 of sketch 3 contours L0 A1 L1 A2 | L3 A3 A4 L4 bodies 20 21 22
fillet "모깎기8" radius 0.1 24 edges at (107.25, 151, 94.5) (105.75, 151, 95) (107.25, 151, 95.5) (108.75, 151, 95) (102.75, 151, 94.5) (101.25, 151, 95) (102.75, 151, 95.5) (104.25, 151, 95) (97.25, 151, 65.5) (98.75, 151, 65) (97.25, 151, 64.5) (95.75, 151, 65) (92.75, 151, 65.5) (94.25, 151, 65) (92.75, 151, 64.5) (91.25, 151, 65) (87.25, 151, 34.5) (85.75, 151, 35) (87.25, 151, 35.5) (88.75, 151, 35) (82.75, 151, 34.5) (81.25, 151, 35) (82.75, 151, 35.5) (84.25, 151, 35) on bodies 20 21 22
copy_body "CopyPasteBodies17" bodies 27 makes body 29
move_body "이동23" bodies 29 to x (1, 0, 0) y (0, 1, 0) z (0, 0, 1) at (35, 0, 0)
copy_body "CopyPasteBodies18" bodies 29 makes body 30
move_body "이동24" bodies 30 to x (1, 0, 0) y (0, 1, 0) z (0, 0, 1) at (10, 0, 30)
copy_body "CopyPasteBodies19" bodies 30 makes body 31
move_body "이동25" bodies 31 to x (1, 0, 0) y (0, 1, 0) z (0, 0, 1) at (10, 0, 30)
move_body "이동26" bodies 31 to x (-1, 0, 0) y (0, 1, 0) z (0, 0, -1) at (210, 0, 190.0089)
copy_body "CopyPasteBodies20" bodies 28 makes body 32
move_body "이동27" bodies 32 to x (1, 0, 0) y (0, 1, 0) z (0, 0, 1) at (35, 0, 0)
copy_body "CopyPasteBodies21" bodies 32 makes body 33
move_body "이동28" bodies 33 to x (1, 0, 0) y (0, 1, 0) z (0, 0, 1) at (10, 0, 30)
copy_body "CopyPasteBodies22" bodies 33 makes body 34
move_body "이동29" bodies 34 to x (1, 0, 0) y (0, 1, 0) z (0, 0, 1) at (10, 0, 30)
move_body "이동30" bodies 33 to x (-1, 0, 0) y (0, 1, 0) z (0, 0, -1) at (190, 0, 130.0089)
combine "결합5" operation add target body 19 tool bodies 28 27
combine "결합6" operation add target body 20 tool bodies 31 34
combine "결합7" operation add target body 21 tool bodies 33 30
combine "결합8" operation add target body 22 tool bodies 29 32
loft "로프트1" add section 1 face at (29.67, 2.8887, 93.0045) section 2 face at (40.316, 2.8681, 67.0045) on bodies 17 18 bodies 17 18
loft "로프트2" add section 1 face at (40.316, 152.1319, 63.0045) section 2 face at (49.684, 152.1319, 37.0045) on bodies 17 19 bodies 17 19
loft "로프트3" add section 1 face at (104.684, 2.8681, 93.0045) section 2 face at (95.316, 2.8681, 67.0045) on bodies 20 21 bodies 20 21
loft "로프트4" add section 1 face at (95.316, 152.1319, 63.0045) section 2 face at (84.684, 152.1319, 37.0045) on bodies 20 22 bodies 20 22
sketch "스케치24" plane through (0, 0, 5) normal (0, 0, 1) x (-1, 0, 0)
  line L0 (-5, -155) -> (-5, -150)
  line L1 (-5, -150) -> (-130, -150)
  line L2 (-130, -150) -> (-130, -155)
  line L3 (-130, -155) -> (-5, -155)
  line L4 (-67.5, -155) -> (-65, -155)
  line L5 (-65, -155) -> (-65, -150)
  line L6 (-65, -150) -> (-70, -150)
  line L7 (-70, -150) -> (-70, -155)
  dimension "d344" = 2.5
  dimension "d345" = 90
  dimension "d346" = 5
  constraint midpoint L3 L4.start
  constraint parallel L3 L4
  constraint coincident L1 L5.end
  constraint perpendicular L1 L5
  constraint coincident L3 L7.end
  constraint perpendicular L3 L7
  measures "d344" distance of L4.start L4.end
  measures "d345" angle of L5 L6
  measures "d346" distance of L5.end L6.end
extrude "돌출62" add sketch "스케치24" along normal blind 125 contours L1 L3 L4 L5 L6 L7 bodies 1
